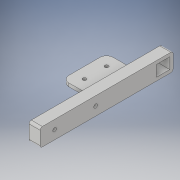
# Autodesk Inventor part: Wheel IR Holder LH
Saved by Autodesk Inventor 2018 (Build 220112000, 112)
## iProperties
Created: 2018-05-01
Part Number: Wheel IR Holder LH
Material: Generic
Document SubType Name: Modeling
Designer: alexs
Density: 1 g/cm^3
Appearance: Default
Author: alexs
Autodesk Inventor part; units mm, degrees
ref_plane "YZ Plane" through (0, 0, 0) normal (1, 0, 0) x (0, 1, 0)
ref_plane "XZ Plane" through (0, 0, 0) normal (0, 1, 0) x (-1, 0, 0)
ref_plane "XY Plane" through (0, 0, 0) normal (0, 0, 1) x (1, 0, 0)
sketch "Sketch1" plane through (0, 0, 0) normal (1, 0, 0) x (0, 1, 0)
  line L0 (0, 0) -> (12, 0)
  line L1 (12, 0) -> (12, 10)
  line L2 (12, 10) -> (0, 10)
  line L3 (0, 10) -> (0, 0)
  line L4 (-105, -3) -> (15, -3)
  line L5 (15, -3) -> (15, 13)
  line L6 (15, 13) -> (-105, 13)
  line L7 (-105, 13) -> (-105, -3)
  point P0 (0, 5)
  dimension "d0" = 12
  dimension "d1" = 10
  dimension "d4" = 16
  dimension "d5" = 3
  dimension "d6" = 120
  dimension "d7" = 3
  constraints: 16 end point, 4 parallel, 2 horizontal, 2 perpendicular, 1 midpoint
  measures "d0" distance of L2.end L1.end
  measures "d1" distance of L1.end L0.end
  measures "d4" distance of L4.end L5.end
  measures "d5" distance between parallel lines of L4 L0
  measures "d6" distance of L5.end L6.end
  measures "d7" distance between parallel lines of L5 L1
extrude "Extrusion1" add sketch "Sketch1" along normal blind 10
sketch "Sketch2" plane through (10, 0, 0) normal (1, 0, 0) x (0, 0, -1)
  circle A0 centre (-5, -92) radius 1.6
  circle A1 centre (-5, -55) radius 1.6
  line L0 (0, 0) -> (-10, 0) projected
  line L1 (3, -105) -> (3, 15) projected
  dimension "d14" = 3.2
  dimension "d15" = 3.2
  dimension "d16" = 55
  dimension "d17" = 37
  dimension "d18" = 8
  dimension "d19" = 8
  constraints: 2 centre point
  measures "d14" diameter of A0
  measures "d15" diameter of A1
  measures "d16" distance from line of A1.centre L0
  measures "d17" distance between centres of A0 A1
  measures "d18" distance from line of L1 A0.centre
  measures "d19" distance from line of L1 A1.centre
extrude "Extrusion2" cut sketch "Sketch2" against normal blind 6
sketch "Sketch3" plane through (0, 0, 0) normal (-1, 0, 0) x (0, 0, 1)
  line L0 (10, 0) -> (0, 0) construction
  line L1 (8, -15) -> (11, -15)
  line L2 (11, -15) -> (11, -55)
  line L3 (11, -55) -> (8, -55)
  line L4 (8, -55) -> (8, -15)
  line L5 (13, 15) -> (13, -105) projected
  line L6 (-3, 15) -> (13, 15) projected
  dimension "d22" = 3
  dimension "d23" = 40
  dimension "d24" = 2
  dimension "d25" = 30
  constraints: 8 end point, 2 parallel, 1 horizontal, 1 perpendicular
  measures "d22" distance of L2.end L3.end
  measures "d23" distance of L1.end L2.end
  measures "d24" distance between parallel lines of L5 L2
  measures "d25" distance between parallel lines of L6 L1
extrude "Extrusion4" add sketch "Sketch3" along normal blind 20
fillet "Fillet2" radius 6 2 edges at (-20, -55, 9.5) (-20, -15, 9.5)
sketch "Sketch4" plane through (0, -55, 11) normal (0, 0, 1) x (1, 0, 0)
  circle A0 centre (-10, 10) radius 1.6
  circle A1 centre (-10, 30) radius 1.6
  line L0 (0, 70) -> (0, -50) projected
  line L1 (0, 0) -> (-14, 0) projected
  line L2 (0, 40) -> (-14, 40) projected
  point P0 (0, 55)
  dimension "d35" = 3.2
  dimension "d36" = 3.2
  dimension "d37" = 10
  dimension "d38" = 10
  dimension "d39" = 10
  dimension "d40" = 10
  constraints: 2 centre point
  measures "d35" diameter of A0
  measures "d36" diameter of A1
  measures "d37" distance from line of L0 A0.centre
  measures "d38" distance from line of L0 A1.centre
  measures "d39" distance from line of L1 A0.centre
  measures "d40" distance from line of L2 A1.centre
fillet "Fillet3" radius 2 4 edges at (5, -105, 13) (5, 15, 13) (5, 15, -3) (5, -105, -3)
extrude "Extrusion5" cut sketch "Sketch4" against normal through all
equation "\"d5\" = -0.5 * d1 + 0.5 * d4"
equation "\"d7\" = d5"
equation "\"d19\" = d18"
equation "\"d38\" = d37"
equation "\"d40\" = d39"
body "Solid1"
